Autodesk Inventor part; units mm, degrees
(part 4 of 6)
  line L2681 (34.7928, 6.3295) -> (34.8431, 6.2385)
  line L2682 (34.8431, 6.2385) -> (34.8956, 6.1628)
  line L2683 (34.8956, 6.1628) -> (34.9493, 6.1023)
  line L2684 (34.9493, 6.1023) -> (35.003, 6.0571)
  line L2685 (35.003, 6.0571) -> (35.0554, 6.0269)
  line L2686 (35.0554, 6.0269) -> (35.0808, 6.0175)
  line L2687 (35.0808, 6.0175) -> (35.1054, 6.0117)
  line L2688 (35.1054, 6.0117) -> (35.1292, 6.0095)
  line L2689 (35.1292, 6.0095) -> (35.1519, 6.011)
  line L2690 (35.1519, 6.011) -> (35.1787, 6.0178)
  line L2691 (35.1787, 6.0178) -> (35.427, 6.1078)
  line L2692 (35.427, 6.1078) -> (35.5068, 6.1343)
  line L2693 (35.5068, 6.1343) -> (35.587, 6.1598)
  line L2694 (35.587, 6.1598) -> (35.8408, 6.2329)
  line L2695 (35.8408, 6.2329) -> (35.8665, 6.2431)
  line L2696 (35.8665, 6.2431) -> (35.8857, 6.2553)
  line L2697 (35.8857, 6.2553) -> (35.9037, 6.271)
  line L2698 (35.9037, 6.271) -> (35.9202, 6.2902)
  line L2699 (35.9202, 6.2902) -> (35.9352, 6.3128)
  line L2700 (35.9352, 6.3128) -> (35.9599, 6.368)
  line L2701 (35.9599, 6.368) -> (35.9767, 6.4361)
  line L2702 (35.9767, 6.4361) -> (35.9846, 6.5166)
  line L2703 (35.9846, 6.5166) -> (35.9826, 6.6088)
  line L2704 (35.9826, 6.6088) -> (35.9698, 6.7119)
  line L2705 (35.9698, 6.7119) -> (35.9451, 6.8253)
  line L2706 (35.9451, 6.8253) -> (35.9303, 6.8806)
  line L2707 (35.9303, 6.8806) -> (35.9204, 6.982)
  line L2708 (35.9204, 6.982) -> (35.9201, 7.1118)
  line L2709 (35.9201, 7.1118) -> (35.925, 7.1945)
  line L2710 (35.925, 7.1945) -> (35.9346, 7.2899)
  line L2711 (35.9346, 7.2899) -> (35.9499, 7.3968)
  line L2712 (35.9499, 7.3968) -> (35.9719, 7.5149)
  line L2713 (35.9719, 7.5149) -> (36.0023, 7.6468)
  line L2714 (36.0023, 7.6468) -> (36.0404, 7.7856)
  line L2715 (36.0404, 7.7856) -> (36.0885, 7.9358)
  line L2716 (36.0885, 7.9358) -> (36.147, 8.0951)
  line L2717 (36.147, 8.0951) -> (36.217, 8.2637)
  line L2718 (36.217, 8.2637) -> (36.286, 8.4128)
  arc A83 (36.9384, 8.4814) -> (36.286, 8.4128) centre (37.5, 0) ccw
  line L2719 (36.9384, 8.4814) -> (37.0368, 8.3499)
  line L2720 (37.0368, 8.3499) -> (37.1404, 8.1995)
  line L2721 (37.1404, 8.1995) -> (37.2307, 8.0558)
  line L2722 (37.2307, 8.0558) -> (37.309, 7.919)
  line L2723 (37.309, 7.919) -> (37.3751, 7.7911)
  line L2724 (37.3751, 7.7911) -> (37.4323, 7.6684)
  line L2725 (37.4323, 7.6684) -> (37.4783, 7.5575)
  line L2726 (37.4783, 7.5575) -> (37.5155, 7.4561)
  line L2727 (37.5155, 7.4561) -> (37.5448, 7.3648)
  line L2728 (37.5448, 7.3648) -> (37.5667, 7.2849)
  line L2729 (37.5667, 7.2849) -> (37.5935, 7.1579)
  line L2730 (37.5935, 7.1579) -> (37.6048, 7.0566)
  line L2731 (37.6048, 7.0566) -> (37.6018, 6.9994)
  line L2732 (37.6018, 6.9994) -> (37.6013, 6.8834)
  line L2733 (37.6013, 6.8834) -> (37.6102, 6.7798)
  line L2734 (37.6102, 6.7798) -> (37.6274, 6.6893)
  line L2735 (37.6274, 6.6893) -> (37.6519, 6.6122)
  line L2736 (37.6519, 6.6122) -> (37.6825, 6.5491)
  line L2737 (37.6825, 6.5491) -> (37.7181, 6.5002)
  line L2738 (37.7181, 6.5002) -> (37.7375, 6.4812)
  line L2739 (37.7375, 6.4812) -> (37.7576, 6.4659)
  line L2740 (37.7576, 6.4659) -> (37.7784, 6.4543)
  line L2741 (37.7784, 6.4543) -> (37.7998, 6.4463)
  line L2742 (37.7998, 6.4463) -> (37.8271, 6.4417)
  line L2743 (37.8271, 6.4417) -> (38.0905, 6.4229)
  line L2744 (38.0905, 6.4229) -> (38.1742, 6.4147)
  line L2745 (38.1742, 6.4147) -> (38.2578, 6.4054)
  line L2746 (38.2578, 6.4054) -> (38.5194, 6.3689)
  line L2747 (38.5194, 6.3689) -> (38.547, 6.3678)
  line L2748 (38.547, 6.3678) -> (38.5696, 6.3711)
  line L2749 (38.5696, 6.3711) -> (38.5923, 6.3781)
  line L2750 (38.5923, 6.3781) -> (38.6152, 6.3889)
  line L2751 (38.6152, 6.3889) -> (38.6381, 6.4035)
  line L2752 (38.6381, 6.4035) -> (38.6831, 6.4439)
  line L2753 (38.6831, 6.4439) -> (38.7262, 6.4993)
  line L2754 (38.7262, 6.4993) -> (38.7661, 6.5696)
  line L2755 (38.7661, 6.5696) -> (38.8018, 6.6546)
  line L2756 (38.8018, 6.6546) -> (38.832, 6.754)
  line L2757 (38.832, 6.754) -> (38.8557, 6.8676)
  line L2758 (38.8557, 6.8676) -> (38.8646, 6.9242)
  line L2759 (38.8646, 6.9242) -> (38.8968, 7.0209)
  line L2760 (38.8968, 7.0209) -> (38.9493, 7.1396)
  line L2761 (38.9493, 7.1396) -> (38.9874, 7.2131)
  line L2762 (38.9874, 7.2131) -> (39.035, 7.2964)
  line L2763 (39.035, 7.2964) -> (39.0925, 7.3878)
  line L2764 (39.0925, 7.3878) -> (39.1606, 7.4867)
  line L2765 (39.1606, 7.4867) -> (39.242, 7.5949)
  line L2766 (39.242, 7.5949) -> (39.3333, 7.7062)
  line L2767 (39.3333, 7.7062) -> (39.4383, 7.8238)
  line L2768 (39.4383, 7.8238) -> (39.5565, 7.9456)
  line L2769 (39.5565, 7.9456) -> (39.6891, 8.0711)
  line L2770 (39.6891, 8.0711) -> (39.8127, 8.1793)
  arc A84 (40.4366, 7.9766) -> (39.8127, 8.1793) centre (37.5, 0) ccw
  line L2771 (40.4366, 7.9766) -> (40.4731, 7.8164)
  line L2772 (40.4731, 7.8164) -> (40.5065, 7.6369)
  line L2773 (40.5065, 7.6369) -> (40.5306, 7.4689)
  line L2774 (40.5306, 7.4689) -> (40.5464, 7.312)
  line L2775 (40.5464, 7.312) -> (40.5549, 7.1683)
  line L2776 (40.5549, 7.1683) -> (40.5571, 7.033)
  line L2777 (40.5571, 7.033) -> (40.5541, 6.9129)
  line L2778 (40.5541, 6.9129) -> (40.5468, 6.8051)
  line L2779 (40.5468, 6.8051) -> (40.5364, 6.7098)
  line L2780 (40.5364, 6.7098) -> (40.524, 6.628)
  line L2781 (40.524, 6.628) -> (40.4968, 6.501)
  line L2782 (40.4968, 6.501) -> (40.466, 6.4039)
  line L2783 (40.466, 6.4039) -> (40.4399, 6.3528)
  line L2784 (40.4399, 6.3528) -> (40.3923, 6.2471)
  line L2785 (40.3923, 6.2471) -> (40.3583, 6.1489)
  line L2786 (40.3583, 6.1489) -> (40.3372, 6.0591)
  line L2787 (40.3372, 6.0591) -> (40.3282, 5.9788)
  line L2788 (40.3282, 5.9788) -> (40.3305, 5.9086)
  line L2789 (40.3305, 5.9086) -> (40.3431, 5.8495)
  line L2790 (40.3431, 5.8495) -> (40.3531, 5.8243)
  line L2791 (40.3531, 5.8243) -> (40.3653, 5.8021)
  line L2792 (40.3653, 5.8021) -> (40.3796, 5.783)
  line L2793 (40.3796, 5.783) -> (40.3959, 5.7671)
  line L2794 (40.3959, 5.7671) -> (40.4189, 5.7518)
  line L2795 (40.4189, 5.7518) -> (40.6519, 5.6274)
  line L2796 (40.6519, 5.6274) -> (40.725, 5.5859)
  line L2797 (40.725, 5.5859) -> (40.7976, 5.5434)
  line L2798 (40.7976, 5.5434) -> (41.0218, 5.4037)
  line L2799 (41.0218, 5.4037) -> (41.0465, 5.3914)
  line L2800 (41.0465, 5.3914) -> (41.0684, 5.3853)
  line L2801 (41.0684, 5.3853) -> (41.0921, 5.3824)
  line L2802 (41.0921, 5.3824) -> (41.1174, 5.383)
  line L2803 (41.1174, 5.383) -> (41.1443, 5.387)
  line L2804 (41.1443, 5.387) -> (41.2018, 5.4056)
  line L2805 (41.2018, 5.4056) -> (41.2637, 5.4387)
  line L2806 (41.2637, 5.4387) -> (41.3288, 5.4866)
  line L2807 (41.3288, 5.4866) -> (41.3959, 5.5498)
  line L2808 (41.3959, 5.5498) -> (41.464, 5.6283)
  line L2809 (41.464, 5.6283) -> (41.5318, 5.7225)
  line L2810 (41.5318, 5.7225) -> (41.563, 5.7705)
  line L2811 (41.563, 5.7705) -> (41.6317, 5.8458)
  line L2812 (41.6317, 5.8458) -> (41.728, 5.9328)
  line L2813 (41.728, 5.9328) -> (41.7927, 5.9845)
  line L2814 (41.7927, 5.9845) -> (41.87, 6.0412)
  line L2815 (41.87, 6.0412) -> (41.9597, 6.1014)
  line L2816 (41.9597, 6.1014) -> (42.0622, 6.1641)
  line L2817 (42.0622, 6.1641) -> (42.1805, 6.2298)
  line L2818 (42.1805, 6.2298) -> (42.3092, 6.2943)
  line L2819 (42.3092, 6.2943) -> (42.453, 6.359)
  line L2820 (42.453, 6.359) -> (42.6105, 6.4222)
  line L2821 (42.6105, 6.4222) -> (42.7827, 6.4829)
  line L2822 (42.7827, 6.4829) -> (42.9396, 6.5315)
  arc A85 (43.4271, 6.0925) -> (42.9396, 6.5315) centre (37.5, 0) ccw
  line L2823 (43.4271, 6.0925) -> (43.3952, 5.9314)
  line L2824 (43.3952, 5.9314) -> (43.3528, 5.7538)
  line L2825 (43.3528, 5.7538) -> (43.3065, 5.5905)
  line L2826 (43.3065, 5.5905) -> (43.2571, 5.4408)
  line L2827 (43.2571, 5.4408) -> (43.2064, 5.3061)
  line L2828 (43.2064, 5.3061) -> (43.1534, 5.1815)
  line L2829 (43.1534, 5.1815) -> (43.1018, 5.073)
  line L2830 (43.1018, 5.073) -> (43.0513, 4.9775)
  line L2831 (43.0513, 4.9775) -> (43.003, 4.8947)
  line L2832 (43.003, 4.8947) -> (42.9584, 4.825)
  line L2833 (42.9584, 4.825) -> (42.8819, 4.7201)
  line L2834 (42.8819, 4.7201) -> (42.8142, 4.6439)
  line L2835 (42.8142, 4.6439) -> (42.7697, 4.6078)
  line L2836 (42.7697, 4.6078) -> (42.6832, 4.5306)
  line L2837 (42.6832, 4.5306) -> (42.6121, 4.4547)
  line L2838 (42.6121, 4.4547) -> (42.5564, 4.3813)
  line L2839 (42.5564, 4.3813) -> (42.5155, 4.3115)
  line L2840 (42.5155, 4.3115) -> (42.489, 4.2466)
  line L2841 (42.489, 4.2466) -> (42.4765, 4.1874)
  line L2842 (42.4765, 4.1874) -> (42.4754, 4.1603)
  line L2843 (42.4754, 4.1603) -> (42.4775, 4.1351)
  line L2844 (42.4775, 4.1351) -> (42.4828, 4.1118)
  line L2845 (42.4828, 4.1118) -> (42.4912, 4.0906)
  line L2846 (42.4912, 4.0906) -> (42.506, 4.0673)
  line L2847 (42.506, 4.0673) -> (42.6683, 3.8589)
  line L2848 (42.6683, 3.8589) -> (42.7182, 3.7912)
  line L2849 (42.7182, 3.7912) -> (42.7672, 3.7229)
  line L2850 (42.7672, 3.7229) -> (42.9152, 3.5041)
  line L2851 (42.9152, 3.5041) -> (42.9328, 3.4828)
  line L2852 (42.9328, 3.4828) -> (42.9503, 3.4683)
  line L2853 (42.9503, 3.4683) -> (42.9708, 3.456)
  line L2854 (42.9708, 3.456) -> (42.9942, 3.4462)
  line L2855 (42.9942, 3.4462) -> (43.0203, 3.439)
  line L2856 (43.0203, 3.439) -> (43.0804, 3.4326)
  line L2857 (43.0804, 3.4326) -> (43.1504, 3.4376)
  line L2858 (43.1504, 3.4376) -> (43.2294, 3.455)
  line L2859 (43.2294, 3.455) -> (43.3164, 3.4854)
  line L2860 (43.3164, 3.4854) -> (43.4105, 3.5294)
  line L2861 (43.4105, 3.5294) -> (43.5107, 3.5879)
  line L2862 (43.5107, 3.5879) -> (43.5588, 3.6191)
  line L2863 (43.5588, 3.6191) -> (43.6522, 3.6599)
  line L2864 (43.6522, 3.6599) -> (43.7755, 3.7002)
  line L2865 (43.7755, 3.7002) -> (43.8557, 3.7212)
  line L2866 (43.8557, 3.7212) -> (43.9494, 3.7415)
  line L2867 (43.9494, 3.7415) -> (44.0558, 3.76)
  line L2868 (44.0558, 3.76) -> (44.1749, 3.7755)
  line L2869 (44.1749, 3.7755) -> (44.3097, 3.7874)
  line L2870 (44.3097, 3.7874) -> (44.4536, 3.794)
  line L2871 (44.4536, 3.794) -> (44.6112, 3.7947)
  line L2872 (44.6112, 3.7947) -> (44.7808, 3.7883)
  line L2873 (44.7808, 3.7883) -> (44.9628, 3.7738)
  line L2874 (44.9628, 3.7738) -> (45.1259, 3.7543)
  arc A86 (45.3927, 3.155) -> (45.1259, 3.7543) centre (37.5, 0) ccw
  line L2875 (45.3927, 3.155) -> (45.2981, 3.0208)
  line L2876 (45.2981, 3.0208) -> (45.1871, 2.8758)
  line L2877 (45.1871, 2.8758) -> (45.0783, 2.7455)
  line L2878 (45.0783, 2.7455) -> (44.9724, 2.6288)
  line L2879 (44.9724, 2.6288) -> (44.8712, 2.5263)
  line L2880 (44.8712, 2.5263) -> (44.7722, 2.4341)
  line L2881 (44.7722, 2.4341) -> (44.6809, 2.356)
  line L2882 (44.6809, 2.356) -> (44.5959, 2.2893)
  line L2883 (44.5959, 2.2893) -> (44.5181, 2.2332)
  line L2884 (44.5181, 2.2332) -> (44.449, 2.1877)
  line L2885 (44.449, 2.1877) -> (44.3364, 2.123)
  line L2886 (44.3364, 2.123) -> (44.2436, 2.0809)
  line L2887 (44.2436, 2.0809) -> (44.1883, 2.0661)
  line L2888 (44.1883, 2.0661) -> (44.0778, 2.0307)
  line L2889 (44.0778, 2.0307) -> (43.9821, 1.9903)
  line L2890 (43.9821, 1.9903) -> (43.9013, 1.9459)
  line L2891 (43.9013, 1.9459) -> (43.8355, 1.8988)
  line L2892 (43.8355, 1.8988) -> (43.7849, 1.8502)
  line L2893 (43.7849, 1.8502) -> (43.7494, 1.8012)
  line L2894 (43.7494, 1.8012) -> (43.7374, 1.777)
  line L2895 (43.7374, 1.777) -> (43.729, 1.7531)
  line L2896 (43.729, 1.7531) -> (43.7244, 1.7297)
  line L2897 (43.7244, 1.7297) -> (43.7235, 1.7069)
  line L2898 (43.7235, 1.7069) -> (43.7275, 1.6796)
  line L2899 (43.7275, 1.6796) -> (43.7911, 1.4232)
  line L2900 (43.7911, 1.4232) -> (43.8091, 1.341)
  line L2901 (43.8091, 1.341) -> (43.826, 1.2587)
  line L2902 (43.826, 1.2587) -> (43.8722, 0.9986)
  line L2903 (43.8722, 0.9986) -> (43.8797, 0.972)
  line L2904 (43.8797, 0.972) -> (43.8898, 0.9516)
  line L2905 (43.8898, 0.9516) -> (43.9035, 0.9321)
  line L2906 (43.9035, 0.9321) -> (43.9209, 0.9136)
  line L2907 (43.9209, 0.9136) -> (43.9418, 0.8964)
  line L2908 (43.9418, 0.8964) -> (43.9941, 0.8661)
  line L2909 (43.9941, 0.8661) -> (44.0601, 0.8422)
  line L2910 (44.0601, 0.8422) -> (44.1393, 0.8259)
  line L2911 (44.1393, 0.8259) -> (44.2312, 0.8183)
  line L2912 (44.2312, 0.8183) -> (44.3351, 0.8203)
  line L2913 (44.3351, 0.8203) -> (44.4504, 0.8329)
  line L2914 (44.4504, 0.8329) -> (44.507, 0.8419)
  line L2915 (44.507, 0.8419) -> (44.6089, 0.8412)
  line L2916 (44.6089, 0.8412) -> (44.738, 0.8278)
  line L2917 (44.738, 0.8278) -> (44.8197, 0.8144)
  line L2918 (44.8197, 0.8144) -> (44.9136, 0.7948)
  line L2919 (44.9136, 0.7948) -> (45.0183, 0.7684)
  line L2920 (45.0183, 0.7684) -> (45.1335, 0.7342)
  line L2921 (45.1335, 0.7342) -> (45.2615, 0.6902)
  line L2922 (45.2615, 0.6902) -> (45.3956, 0.6378)
  line L2923 (45.3956, 0.6378) -> (45.5398, 0.5742)
  line L2924 (45.5398, 0.5742) -> (45.6922, 0.4994)
  line L2925 (45.6922, 0.4994) -> (45.8526, 0.4122)
  line L2926 (45.8526, 0.4122) -> (45.9936, 0.328)
  arc A87 (45.9936, -0.328) -> (45.9936, 0.328) centre (37.5, 0) ccw
  line L2927 (45.9936, -0.328) -> (45.8526, -0.4122)
  line L2928 (45.8526, -0.4122) -> (45.6922, -0.4994)
  line L2929 (45.6922, -0.4994) -> (45.5398, -0.5742)
  line L2930 (45.5398, -0.5742) -> (45.3956, -0.6378)
  line L2931 (45.3956, -0.6378) -> (45.2615, -0.6902)
  line L2932 (45.2615, -0.6902) -> (45.1335, -0.7342)
  line L2933 (45.1335, -0.7342) -> (45.0183, -0.7684)
  line L2934 (45.0183, -0.7684) -> (44.9136, -0.7948)
  line L2935 (44.9136, -0.7948) -> (44.8197, -0.8144)
  line L2936 (44.8197, -0.8144) -> (44.738, -0.8278)
  line L2937 (44.738, -0.8278) -> (44.6089, -0.8412)
  line L2938 (44.6089, -0.8412) -> (44.507, -0.8419)
  line L2939 (44.507, -0.8419) -> (44.4504, -0.8329)
  line L2940 (44.4504, -0.8329) -> (44.3351, -0.8203)
  line L2941 (44.3351, -0.8203) -> (44.2312, -0.8183)
  line L2942 (44.2312, -0.8183) -> (44.1393, -0.8259)
  line L2943 (44.1393, -0.8259) -> (44.0601, -0.8422)
  line L2944 (44.0601, -0.8422) -> (43.9941, -0.8661)
  line L2945 (43.9941, -0.8661) -> (43.9418, -0.8964)
  line L2946 (43.9418, -0.8964) -> (43.9209, -0.9136)
  line L2947 (43.9209, -0.9136) -> (43.9035, -0.9321)
  line L2948 (43.9035, -0.9321) -> (43.8898, -0.9516)
  line L2949 (43.8898, -0.9516) -> (43.8797, -0.972)
  line L2950 (43.8797, -0.972) -> (43.8722, -0.9986)
  line L2951 (43.8722, -0.9986) -> (43.826, -1.2587)
  line L2952 (43.826, -1.2587) -> (43.8091, -1.341)
  line L2953 (43.8091, -1.341) -> (43.7911, -1.4232)
  line L2954 (43.7911, -1.4232) -> (43.7275, -1.6796)
  line L2955 (43.7275, -1.6796) -> (43.7235, -1.7069)
  line L2956 (43.7235, -1.7069) -> (43.7244, -1.7297)
  line L2957 (43.7244, -1.7297) -> (43.729, -1.7531)
  line L2958 (43.729, -1.7531) -> (43.7374, -1.777)
  line L2959 (43.7374, -1.777) -> (43.7494, -1.8012)
  line L2960 (43.7494, -1.8012) -> (43.7849, -1.8502)
  line L2961 (43.7849, -1.8502) -> (43.8355, -1.8988)
  line L2962 (43.8355, -1.8988) -> (43.9013, -1.9459)
  line L2963 (43.9013, -1.9459) -> (43.9821, -1.9903)
  line L2964 (43.9821, -1.9903) -> (44.0778, -2.0307)
  line L2965 (44.0778, -2.0307) -> (44.1883, -2.0661)
  line L2966 (44.1883, -2.0661) -> (44.2436, -2.0809)
  line L2967 (44.2436, -2.0809) -> (44.3364, -2.123)
  line L2968 (44.3364, -2.123) -> (44.449, -2.1877)
  line L2969 (44.449, -2.1877) -> (44.5181, -2.2332)
  line L2970 (44.5181, -2.2332) -> (44.5959, -2.2893)
  line L2971 (44.5959, -2.2893) -> (44.6809, -2.356)
  line L2972 (44.6809, -2.356) -> (44.7722, -2.4341)
  line L2973 (44.7722, -2.4341) -> (44.8712, -2.5263)
  line L2974 (44.8712, -2.5263) -> (44.9724, -2.6288)
  line L2975 (44.9724, -2.6288) -> (45.0783, -2.7455)
  line L2976 (45.0783, -2.7455) -> (45.1871, -2.8758)
  line L2977 (45.1871, -2.8758) -> (45.2981, -3.0208)
  line L2978 (45.2981, -3.0208) -> (45.3927, -3.155)
  arc A88 (45.1259, -3.7543) -> (45.3927, -3.155) centre (37.5, 0) ccw
  line L2979 (45.1259, -3.7543) -> (44.9628, -3.7738)
  line L2980 (44.9628, -3.7738) -> (44.7808, -3.7883)
  line L2981 (44.7808, -3.7883) -> (44.6112, -3.7947)
  line L2982 (44.6112, -3.7947) -> (44.4536, -3.794)
  line L2983 (44.4536, -3.794) -> (44.3097, -3.7874)
  line L2984 (44.3097, -3.7874) -> (44.1749, -3.7755)
  line L2985 (44.1749, -3.7755) -> (44.0558, -3.76)
  line L2986 (44.0558, -3.76) -> (43.9494, -3.7415)
  line L2987 (43.9494, -3.7415) -> (43.8557, -3.7212)
  line L2988 (43.8557, -3.7212) -> (43.7755, -3.7002)
  line L2989 (43.7755, -3.7002) -> (43.6522, -3.6599)
  line L2990 (43.6522, -3.6599) -> (43.5588, -3.6191)
  line L2991 (43.5588, -3.6191) -> (43.5107, -3.5879)
  line L2992 (43.5107, -3.5879) -> (43.4105, -3.5294)
  line L2993 (43.4105, -3.5294) -> (43.3164, -3.4854)
  line L2994 (43.3164, -3.4854) -> (43.2294, -3.455)
  line L2995 (43.2294, -3.455) -> (43.1504, -3.4376)
  line L2996 (43.1504, -3.4376) -> (43.0804, -3.4326)
  line L2997 (43.0804, -3.4326) -> (43.0203, -3.439)
  line L2998 (43.0203, -3.439) -> (42.9942, -3.4462)
  line L2999 (42.9942, -3.4462) -> (42.9708, -3.456)
  line L3000 (42.9708, -3.456) -> (42.9503, -3.4683)
  line L3001 (42.9503, -3.4683) -> (42.9328, -3.4828)
  line L3002 (42.9328, -3.4828) -> (42.9152, -3.5041)
  line L3003 (42.9152, -3.5041) -> (42.7672, -3.7229)
  line L3004 (42.7672, -3.7229) -> (42.7182, -3.7912)
  line L3005 (42.7182, -3.7912) -> (42.6683, -3.8589)
  line L3006 (42.6683, -3.8589) -> (42.506, -4.0673)
  line L3007 (42.506, -4.0673) -> (42.4912, -4.0906)
  line L3008 (42.4912, -4.0906) -> (42.4828, -4.1118)
  line L3009 (42.4828, -4.1118) -> (42.4775, -4.1351)
  line L3010 (42.4775, -4.1351) -> (42.4754, -4.1603)
  line L3011 (42.4754, -4.1603) -> (42.4765, -4.1874)
  line L3012 (42.4765, -4.1874) -> (42.489, -4.2466)
  line L3013 (42.489, -4.2466) -> (42.5155, -4.3115)
  line L3014 (42.5155, -4.3115) -> (42.5564, -4.3813)
  line L3015 (42.5564, -4.3813) -> (42.6121, -4.4547)
  line L3016 (42.6121, -4.4547) -> (42.6832, -4.5306)
  line L3017 (42.6832, -4.5306) -> (42.7697, -4.6078)
  line L3018 (42.7697, -4.6078) -> (42.8142, -4.6439)
  line L3019 (42.8142, -4.6439) -> (42.8819, -4.7201)
  line L3020 (42.8819, -4.7201) -> (42.9584, -4.825)
  line L3021 (42.9584, -4.825) -> (43.003, -4.8947)
  line L3022 (43.003, -4.8947) -> (43.0513, -4.9775)
  line L3023 (43.0513, -4.9775) -> (43.1018, -5.073)
  line L3024 (43.1018, -5.073) -> (43.1534, -5.1815)
  line L3025 (43.1534, -5.1815) -> (43.2064, -5.3061)
  line L3026 (43.2064, -5.3061) -> (43.2571, -5.4408)
  line L3027 (43.2571, -5.4408) -> (43.3065, -5.5905)
  line L3028 (43.3065, -5.5905) -> (43.3528, -5.7538)
  line L3029 (43.3528, -5.7538) -> (43.3952, -5.9314)
  line L3030 (43.3952, -5.9314) -> (43.4271, -6.0925)
  arc A89 (42.9396, -6.5315) -> (43.4271, -6.0925) centre (37.5, 0) ccw
  line L3031 (42.9396, -6.5315) -> (42.7827, -6.4829)
  line L3032 (42.7827, -6.4829) -> (42.6105, -6.4222)
  line L3033 (42.6105, -6.4222) -> (42.453, -6.359)
  line L3034 (42.453, -6.359) -> (42.3092, -6.2943)
  line L3035 (42.3092, -6.2943) -> (42.1805, -6.2298)
  line L3036 (42.1805, -6.2298) -> (42.0622, -6.1641)
  line L3037 (42.0622, -6.1641) -> (41.9597, -6.1014)
  line L3038 (41.9597, -6.1014) -> (41.87, -6.0412)
  line L3039 (41.87, -6.0412) -> (41.7927, -5.9845)
  line L3040 (41.7927, -5.9845) -> (41.728, -5.9328)
  line L3041 (41.728, -5.9328) -> (41.6317, -5.8458)
  line L3042 (41.6317, -5.8458) -> (41.563, -5.7705)
  line L3043 (41.563, -5.7705) -> (41.5318, -5.7225)
  line L3044 (41.5318, -5.7225) -> (41.464, -5.6283)
  line L3045 (41.464, -5.6283) -> (41.3959, -5.5498)
  line L3046 (41.3959, -5.5498) -> (41.3288, -5.4866)
  line L3047 (41.3288, -5.4866) -> (41.2637, -5.4387)
  line L3048 (41.2637, -5.4387) -> (41.2018, -5.4056)
  line L3049 (41.2018, -5.4056) -> (41.1443, -5.387)
  line L3050 (41.1443, -5.387) -> (41.1174, -5.383)
  line L3051 (41.1174, -5.383) -> (41.0921, -5.3824)
  line L3052 (41.0921, -5.3824) -> (41.0684, -5.3853)
  line L3053 (41.0684, -5.3853) -> (41.0465, -5.3914)
  line L3054 (41.0465, -5.3914) -> (41.0218, -5.4037)
  line L3055 (41.0218, -5.4037) -> (40.7976, -5.5434)
  line L3056 (40.7976, -5.5434) -> (40.725, -5.5859)
  line L3057 (40.725, -5.5859) -> (40.6519, -5.6274)
  line L3058 (40.6519, -5.6274) -> (40.4189, -5.7518)
  line L3059 (40.4189, -5.7518) -> (40.3959, -5.7671)
  line L3060 (40.3959, -5.7671) -> (40.3796, -5.783)
  line L3061 (40.3796, -5.783) -> (40.3653, -5.8021)
  line L3062 (40.3653, -5.8021) -> (40.3531, -5.8243)
  line L3063 (40.3531, -5.8243) -> (40.3431, -5.8495)
  line L3064 (40.3431, -5.8495) -> (40.3305, -5.9086)
  line L3065 (40.3305, -5.9086) -> (40.3282, -5.9788)
  line L3066 (40.3282, -5.9788) -> (40.3372, -6.0591)
  line L3067 (40.3372, -6.0591) -> (40.3583, -6.1489)
  line L3068 (40.3583, -6.1489) -> (40.3923, -6.2471)
  line L3069 (40.3923, -6.2471) -> (40.4399, -6.3528)
  line L3070 (40.4399, -6.3528) -> (40.466, -6.4039)
  line L3071 (40.466, -6.4039) -> (40.4968, -6.501)
  line L3072 (40.4968, -6.501) -> (40.524, -6.628)
  line L3073 (40.524, -6.628) -> (40.5364, -6.7098)
  line L3074 (40.5364, -6.7098) -> (40.5468, -6.8051)
  line L3075 (40.5468, -6.8051) -> (40.5541, -6.9129)
  line L3076 (40.5541, -6.9129) -> (40.5571, -7.033)
  line L3077 (40.5571, -7.033) -> (40.5549, -7.1683)
  line L3078 (40.5549, -7.1683) -> (40.5464, -7.312)
  line L3079 (40.5464, -7.312) -> (40.5306, -7.4689)
  line L3080 (40.5306, -7.4689) -> (40.5065, -7.6369)
  line L3081 (40.5065, -7.6369) -> (40.4731, -7.8164)
  line L3082 (40.4731, -7.8164) -> (40.4366, -7.9766)
  arc A90 (39.8127, -8.1793) -> (40.4366, -7.9766) centre (37.5, 0) ccw
  line L3083 (39.8127, -8.1793) -> (39.6891, -8.0711)
  line L3084 (39.6891, -8.0711) -> (39.5565, -7.9456)
  line L3085 (39.5565, -7.9456) -> (39.4383, -7.8238)
  line L3086 (39.4383, -7.8238) -> (39.3333, -7.7062)
  line L3087 (39.3333, -7.7062) -> (39.242, -7.5949)
  line L3088 (39.242, -7.5949) -> (39.1606, -7.4867)
  line L3089 (39.1606, -7.4867) -> (39.0925, -7.3878)
  line L3090 (39.0925, -7.3878) -> (39.035, -7.2964)
  line L3091 (39.035, -7.2964) -> (38.9874, -7.2131)
  line L3092 (38.9874, -7.2131) -> (38.9493, -7.1396)
  line L3093 (38.9493, -7.1396) -> (38.8968, -7.0209)
  line L3094 (38.8968, -7.0209) -> (38.8646, -6.9242)
  line L3095 (38.8646, -6.9242) -> (38.8557, -6.8676)
  line L3096 (38.8557, -6.8676) -> (38.832, -6.754)
  line L3097 (38.832, -6.754) -> (38.8018, -6.6546)
  line L3098 (38.8018, -6.6546) -> (38.7661, -6.5696)
  line L3099 (38.7661, -6.5696) -> (38.7262, -6.4993)
  line L3100 (38.7262, -6.4993) -> (38.6831, -6.4439)
  line L3101 (38.6831, -6.4439) -> (38.6381, -6.4035)
  line L3102 (38.6381, -6.4035) -> (38.6152, -6.3889)
  line L3103 (38.6152, -6.3889) -> (38.5923, -6.3781)
  line L3104 (38.5923, -6.3781) -> (38.5696, -6.3711)
  line L3105 (38.5696, -6.3711) -> (38.547, -6.3678)
  line L3106 (38.547, -6.3678) -> (38.5194, -6.3689)
  line L3107 (38.5194, -6.3689) -> (38.2578, -6.4054)
  line L3108 (38.2578, -6.4054) -> (38.1742, -6.4147)
  line L3109 (38.1742, -6.4147) -> (38.0905, -6.4229)
  line L3110 (38.0905, -6.4229) -> (37.8271, -6.4417)
  line L3111 (37.8271, -6.4417) -> (37.7998, -6.4463)
  line L3112 (37.7998, -6.4463) -> (37.7784, -6.4543)
  line L3113 (37.7784, -6.4543) -> (37.7576, -6.4659)
  line L3114 (37.7576, -6.4659) -> (37.7375, -6.4812)
  line L3115 (37.7375, -6.4812) -> (37.7181, -6.5002)
  line L3116 (37.7181, -6.5002) -> (37.6825, -6.5491)
  line L3117 (37.6825, -6.5491) -> (37.6519, -6.6122)
  line L3118 (37.6519, -6.6122) -> (37.6274, -6.6893)
  line L3119 (37.6274, -6.6893) -> (37.6102, -6.7798)
  line L3120 (37.6102, -6.7798) -> (37.6013, -6.8834)
  line L3121 (37.6013, -6.8834) -> (37.6018, -6.9994)
  line L3122 (37.6018, -6.9994) -> (37.6048, -7.0566)
  line L3123 (37.6048, -7.0566) -> (37.5935, -7.1579)
  line L3124 (37.5935, -7.1579) -> (37.5667, -7.2849)
  line L3125 (37.5667, -7.2849) -> (37.5448, -7.3648)
  line L3126 (37.5448, -7.3648) -> (37.5155, -7.4561)
  line L3127 (37.5155, -7.4561) -> (37.4783, -7.5575)
  line L3128 (37.4783, -7.5575) -> (37.4323, -7.6684)
  line L3129 (37.4323, -7.6684) -> (37.3751, -7.7911)
  line L3130 (37.3751, -7.7911) -> (37.309, -7.919)
  line L3131 (37.309, -7.919) -> (37.2307, -8.0558)
  line L3132 (37.2307, -8.0558) -> (37.1404, -8.1995)
  line L3133 (37.1404, -8.1995) -> (37.0368, -8.3499)
  line L3134 (37.0368, -8.3499) -> (36.9384, -8.4814)
  arc A91 (36.286, -8.4128) -> (36.9384, -8.4814) centre (37.5, 0) ccw
  line L3135 (36.286, -8.4128) -> (36.217, -8.2637)
  line L3136 (36.217, -8.2637) -> (36.147, -8.0951)
  line L3137 (36.147, -8.0951) -> (36.0885, -7.9358)
  line L3138 (36.0885, -7.9358) -> (36.0404, -7.7856)
  line L3139 (36.0404, -7.7856) -> (36.0023, -7.6468)
  line L3140 (36.0023, -7.6468) -> (35.9719, -7.5149)
  line L3141 (35.9719, -7.5149) -> (35.9499, -7.3968)
  line L3142 (35.9499, -7.3968) -> (35.9346, -7.2899)
  line L3143 (35.9346, -7.2899) -> (35.925, -7.1945)
  line L3144 (35.925, -7.1945) -> (35.9201, -7.1118)
  line L3145 (35.9201, -7.1118) -> (35.9204, -6.982)
  line L3146 (35.9204, -6.982) -> (35.9303, -6.8806)
  line L3147 (35.9303, -6.8806) -> (35.9451, -6.8253)
  line L3148 (35.9451, -6.8253) -> (35.9698, -6.7119)
  line L3149 (35.9698, -6.7119) -> (35.9826, -6.6088)
  line L3150 (35.9826, -6.6088) -> (35.9846, -6.5166)
  line L3151 (35.9846, -6.5166) -> (35.9767, -6.4361)
  line L3152 (35.9767, -6.4361) -> (35.9599, -6.368)
  line L3153 (35.9599, -6.368) -> (35.9352, -6.3128)
  line L3154 (35.9352, -6.3128) -> (35.9202, -6.2902)
  line L3155 (35.9202, -6.2902) -> (35.9037, -6.271)
  line L3156 (35.9037, -6.271) -> (35.8857, -6.2553)
  line L3157 (35.8857, -6.2553) -> (35.8665, -6.2431)
  line L3158 (35.8665, -6.2431) -> (35.8408, -6.2329)
  line L3159 (35.8408, -6.2329) -> (35.587, -6.1598)
  line L3160 (35.587, -6.1598) -> (35.5068, -6.1343)
  line L3161 (35.5068, -6.1343) -> (35.427, -6.1078)
  line L3162 (35.427, -6.1078) -> (35.1787, -6.0178)
  line L3163 (35.1787, -6.0178) -> (35.1519, -6.011)
  line L3164 (35.1519, -6.011) -> (35.1292, -6.0095)
  line L3165 (35.1292, -6.0095) -> (35.1054, -6.0117)
  line L3166 (35.1054, -6.0117) -> (35.0808, -6.0175)
  line L3167 (35.0808, -6.0175) -> (35.0554, -6.0269)
  line L3168 (35.0554, -6.0269) -> (35.003, -6.0571)
  line L3169 (35.003, -6.0571) -> (34.9493, -6.1023)
  line L3170 (34.9493, -6.1023) -> (34.8956, -6.1628)
  line L3171 (34.8956, -6.1628) -> (34.8431, -6.2385)
  line L3172 (34.8431, -6.2385) -> (34.7928, -6.3295)
  line L3173 (34.7928, -6.3295) -> (34.7461, -6.4357)
  line L3174 (34.7461, -6.4357) -> (34.7256, -6.4892)
  line L3175 (34.7256, -6.4892) -> (34.674, -6.5771)
  line L3176 (34.674, -6.5771) -> (34.5979, -6.6822)
  line L3177 (34.5979, -6.6822) -> (34.5454, -6.7463)
  line L3178 (34.5454, -6.7463) -> (34.4815, -6.8178)
  line L3179 (34.4815, -6.8178) -> (34.4063, -6.8953)
  line L3180 (34.4063, -6.8953) -> (34.3191, -6.9779)
  line L3181 (34.3191, -6.9779) -> (34.217, -7.0668)
  line L3182 (34.217, -7.0668) -> (34.1045, -7.1566)
  line L3183 (34.1045, -7.1566) -> (33.9774, -7.2498)
  line L3184 (33.9774, -7.2498) -> (33.8364, -7.3444)
  line L3185 (33.8364, -7.3444) -> (33.6807, -7.4396)
  line L3186 (33.6807, -7.4396) -> (33.5372, -7.5197)
  arc A92 (32.9691, -7.1917) -> (33.5372, -7.5197) centre (37.5, 0) ccw
  line L3187 (32.9691, -7.1917) -> (32.9668, -7.0275)
  line L3188 (32.9668, -7.0275) -> (32.9714, -6.8449)
  line L3189 (32.9714, -6.8449) -> (32.9828, -6.6756)
  line L3190 (32.9828, -6.6756) -> (32.9999, -6.5189)
  line L3191 (32.9999, -6.5189) -> (33.0215, -6.3765)
  line L3192 (33.0215, -6.3765) -> (33.0474, -6.2437)
  line L3193 (33.0474, -6.2437) -> (33.0754, -6.1269)
  line L3194 (33.0754, -6.1269) -> (33.1049, -6.0229)
  line L3195 (33.1049, -6.0229) -> (33.1349, -5.9319)
  line L3196 (33.1349, -5.9319) -> (33.1641, -5.8544)
  line L3197 (33.1641, -5.8544) -> (33.2171, -5.7359)
  line L3198 (33.2171, -5.7359) -> (33.2674, -5.6473)
  line L3199 (33.2674, -5.6473) -> (33.3035, -5.6028)
  line L3200 (33.3035, -5.6028) -> (33.3721, -5.5092)
  line L3201 (33.3721, -5.5092) -> (33.4258, -5.4202)
  line L3202 (33.4258, -5.4202) -> (33.4651, -5.3368)
  line L3203 (33.4651, -5.3368) -> (33.4906, -5.2601)
  line L3204 (33.4906, -5.2601) -> (33.5029, -5.191)
  line L3205 (33.5029, -5.191) -> (33.5028, -5.1306)
  line L3206 (33.5028, -5.1306) -> (33.4983, -5.1038)
  line L3207 (33.4983, -5.1038) -> (33.491, -5.0796)
  line L3208 (33.491, -5.0796) -> (33.481, -5.0579)
  line L3209 (33.481, -5.0579) -> (33.4684, -5.039)
  line L3210 (33.4684, -5.039) -> (33.4491, -5.0192)
  line L3211 (33.4491, -5.0192) -> (33.2469, -4.8492)
  line L3212 (33.2469, -4.8492) -> (33.1841, -4.7933)
  line L3213 (33.1841, -4.7933) -> (33.122, -4.7366)
  line L3214 (33.122, -4.7366) -> (32.9317, -4.5534)
  line L3215 (32.9317, -4.5534) -> (32.9101, -4.5363)
  line L3216 (32.9101, -4.5363) -> (32.8899, -4.5257)
  line L3217 (32.8899, -4.5257) -> (32.8673, -4.518)
  line L3218 (32.8673, -4.518) -> (32.8424, -4.5132)
  line L3219 (32.8424, -4.5132) -> (32.8154, -4.5116)
  line L3220 (32.8154, -4.5116) -> (32.7552, -4.5178)
  line L3221 (32.7552, -4.5178) -> (32.6878, -4.5373)
  line L3222 (32.6878, -4.5373) -> (32.6142, -4.5707)
  line L3223 (32.6142, -4.5707) -> (32.5353, -4.6185)
  line L3224 (32.5353, -4.6185) -> (32.4524, -4.6812)
  line L3225 (32.4524, -4.6812) -> (32.3666, -4.7592)
  line L3226 (32.3666, -4.7592) -> (32.3261, -4.7997)
  line L3227 (32.3261, -4.7997) -> (32.2432, -4.859)
  line L3228 (32.2432, -4.859) -> (32.1309, -4.9241)
  line L3229 (32.1309, -4.9241) -> (32.0569, -4.9613)
  line L3230 (32.0569, -4.9613) -> (31.9695, -5.0006)
  line L3231 (31.9695, -5.0006) -> (31.8692, -5.0408)
  line L3232 (31.8692, -5.0408) -> (31.756, -5.0808)
  line L3233 (31.756, -5.0808) -> (31.6265, -5.1205)
  line L3234 (31.6265, -5.1205) -> (31.4872, -5.1568)
  line L3235 (31.4872, -5.1568) -> (31.3332, -5.1903)
  line L3236 (31.3332, -5.1903) -> (31.1659, -5.2193)
  line L3237 (31.1659, -5.2193) -> (30.9849, -5.243)
  line L3238 (30.9849, -5.243) -> (30.8213, -5.2578)
  arc A93 (30.4357, -4.7271) -> (30.8213, -5.2578) centre (37.5, 0) ccw
  line L3239 (30.4357, -4.7271) -> (30.5004, -4.5761)
  line L3240 (30.676, 2.741) -> (30.453, 2.6211)
  line L3241 (30.453, 2.6211) -> (30.2376, 2.5111)
  line L3242 (30.2376, 2.5111) -> (30.0323, 2.4116)
  line L3243 (30.0323, 2.4116) -> (29.8355, 2.3213)
  line L3244 (29.8355, 2.3213) -> (29.6473, 2.2396)
  line L3245 (29.6473, 2.2396) -> (29.4705, 2.1673)
  line L3246 (29.4705, 2.1673) -> (29.3033, 2.1029)
  line L3247 (29.3033, 2.1029) -> (28.9724, 1.9849)
  line L3248 (28.9724, 1.9849) -> (28.931, 1.9629)
  line L3249 (28.931, 1.9629) -> (28.9033, 1.9404)
  line L3250 (28.9033, 1.9404) -> (28.8892, 1.9178)
  line L3251 (28.8892, 1.9178) -> (28.8876, 1.9012)
  line L3252 (28.8876, 1.9012) -> (28.9103, 1.5151)
  line L3253 (28.9103, 1.5151) -> (28.9281, 1.1288)
  line L3254 (28.9281, 1.1288) -> (28.9314, 1.1124)
  line L3255 (28.9314, 1.1124) -> (28.9478, 1.0915)
  line L3256 (28.9478, 1.0915) -> (28.9777, 1.0719)
  line L3257 (28.9777, 1.0719) -> (29.0211, 1.0544)
  line L3258 (29.0211, 1.0544) -> (29.3626, 0.9717)
  line L3259 (29.3626, 0.9717) -> (29.5356, 0.9251)
  line L3260 (29.5356, 0.9251) -> (29.719, 0.8717)
  line L3261 (29.719, 0.8717) -> (29.9147, 0.8101)
  line L3262 (29.9147, 0.8101) -> (30.1199, 0.7408)
  line L3263 (30.1199, 0.7408) -> (30.3344, 0.6634)
  line L3264 (30.3344, 0.6634) -> (30.5601, 0.5765)
  line L3265 (30.5601, 0.5765) -> (30.7945, 0.4805)
  line L3266 (30.7945, 0.4805) -> (30.9975, 0.3928)
  arc A94 (30.9975, -0.3928) -> (30.9975, 0.3928) centre (0, 0) ccw
  line L3267 (30.9975, -0.3928) -> (30.7945, -0.4805)
  line L3268 (30.7945, -0.4805) -> (30.5601, -0.5765)
  line L3269 (30.5601, -0.5765) -> (30.3344, -0.6634)
  line L3270 (30.3344, -0.6634) -> (30.1199, -0.7408)
  line L3271 (30.1199, -0.7408) -> (29.9147, -0.8101)
  line L3272 (29.9147, -0.8101) -> (29.719, -0.8717)
  line L3273 (29.719, -0.8717) -> (29.5356, -0.9251)
  line L3274 (29.5356, -0.9251) -> (29.3626, -0.9717)
  line L3275 (29.3626, -0.9717) -> (29.0211, -1.0544)
  line L3276 (29.0211, -1.0544) -> (28.9777, -1.0719)
  line L3277 (28.9777, -1.0719) -> (28.9478, -1.0915)
  line L3278 (28.9478, -1.0915) -> (28.9314, -1.1124)
  line L3279 (28.9314, -1.1124) -> (28.9281, -1.1288)
  line L3280 (28.9281, -1.1288) -> (28.9103, -1.5151)
  line L3281 (28.9103, -1.5151) -> (28.8876, -1.9012)
  line L3282 (28.8876, -1.9012) -> (28.8892, -1.9178)
  line L3283 (28.8892, -1.9178) -> (28.9033, -1.9404)
  line L3284 (28.9033, -1.9404) -> (28.931, -1.9629)
  line L3285 (28.931, -1.9629) -> (28.9724, -1.9849)
  line L3286 (28.9724, -1.9849) -> (29.3033, -2.1029)
  line L3287 (29.3033, -2.1029) -> (29.4705, -2.1673)
  line L3288 (29.4705, -2.1673) -> (29.6473, -2.2396)
  line L3289 (29.6473, -2.2396) -> (29.8355, -2.3213)
  line L3290 (29.8355, -2.3213) -> (30.0323, -2.4116)
  line L3291 (30.0323, -2.4116) -> (30.2376, -2.5111)
  line L3292 (30.2376, -2.5111) -> (30.453, -2.6211)
  line L3293 (30.453, -2.6211) -> (30.676, -2.741)
  line L3294 (30.676, -2.741) -> (30.8688, -2.8495)
  arc A95 (30.7866, -3.6308) -> (30.8688, -2.8495) centre (0, 0) ccw
  line L3295 (30.7866, -3.6308) -> (30.5755, -3.6968)
  line L3296 (30.5755, -3.6968) -> (30.3325, -3.7677)
  line L3297 (30.3325, -3.7677) -> (30.0989, -3.8305)
  line L3298 (30.0989, -3.8305) -> (29.8774, -3.8852)
  line L3299 (29.8774, -3.8852) -> (29.6661, -3.9326)
  line L3300 (29.6661, -3.9326) -> (29.465, -3.9734)
  line L3301 (29.465, -3.9734) -> (29.2771, -4.0074)
  line L3302 (29.2771, -4.0074) -> (29.1001, -4.0356)
  line L3303 (29.1001, -4.0356) -> (28.7519, -4.0822)
  line L3304 (28.7519, -4.0822) -> (28.7069, -4.0951)
  line L3305 (28.7069, -4.0951) -> (28.6751, -4.1114)
  line L3306 (28.6751, -4.1114) -> (28.6567, -4.1305)
  line L3307 (28.6567, -4.1305) -> (28.6516, -4.1464)
  line L3308 (28.6516, -4.1464) -> (28.5936, -4.5288)
  line L3309 (28.5936, -4.5288) -> (28.5306, -4.9104)
  line L3310 (28.5306, -4.9104) -> (28.5305, -4.927)
  line L3311 (28.5305, -4.927) -> (28.5421, -4.951)
  line L3312 (28.5421, -4.951) -> (28.5674, -4.9763)
  line L3313 (28.5674, -4.9763) -> (28.6062, -5.0025)
  line L3314 (28.6062, -5.0025) -> (28.9229, -5.1544)
  line L3315 (28.9229, -5.1544) -> (29.0826, -5.2359)
  line L3316 (29.0826, -5.2359) -> (29.2508, -5.3263)
  line L3317 (29.2508, -5.3263) -> (29.4294, -5.4272)
  line L3318 (29.4294, -5.4272) -> (29.6157, -5.5376)
  line L3319 (29.6157, -5.5376) -> (29.8094, -5.658)
  line L3320 (29.8094, -5.658) -> (30.0122, -5.79)
  line L3321 (30.0122, -5.79) -> (30.2214, -5.9325)
  line L3322 (30.2214, -5.9325) -> (30.4018, -6.0605)
  arc A96 (30.2385, -6.829) -> (30.4018, -6.0605) centre (0, 0) ccw
  line L3323 (30.2385, -6.829) -> (30.0216, -6.8726)
  line L3324 (30.0216, -6.8726) -> (29.7725, -6.9177)
  line L3325 (29.7725, -6.9177) -> (29.5336, -6.9557)
  line L3326 (29.5336, -6.9557) -> (29.3077, -6.9869)
  line L3327 (29.3077, -6.9869) -> (29.0926, -7.012)
  line L3328 (29.0926, -7.012) -> (28.8883, -7.0315)
  line L3329 (28.8883, -7.0315) -> (28.6979, -7.0457)
  line L3330 (28.6979, -7.0457) -> (28.5189, -7.0553)
  line L3331 (28.5189, -7.0553) -> (28.1677, -7.0652)
  line L3332 (28.1677, -7.0652) -> (28.1216, -7.0733)
  line L3333 (28.1216, -7.0733) -> (28.0883, -7.0862)
  line L3334 (28.0883, -7.0862) -> (28.0679, -7.1033)
  line L3335 (28.0679, -7.1033) -> (28.0612, -7.1186)
  line L3336 (28.0612, -7.1186) -> (27.9636, -7.4928)
  line L3337 (27.9636, -7.4928) -> (27.861, -7.8657)
  line L3338 (27.861, -7.8657) -> (27.8592, -7.8823)
  line L3339 (27.8592, -7.8823) -> (27.8683, -7.9073)
  line L3340 (27.8683, -7.9073) -> (27.8907, -7.9351)
  line L3341 (27.8907, -7.9351) -> (27.9266, -7.9652)
  line L3342 (27.9266, -7.9652) -> (28.2257, -8.1494)
  line L3343 (28.2257, -8.1494) -> (28.3759, -8.2472)
  line L3344 (28.3759, -8.2472) -> (28.5338, -8.3547)
  line L3345 (28.5338, -8.3547) -> (28.7009, -8.4737)
  line L3346 (28.7009, -8.4737) -> (28.8746, -8.603)
  line L3347 (28.8746, -8.603) -> (29.0547, -8.7429)
  line L3348 (29.0547, -8.7429) -> (29.2425, -8.8954)
  line L3349 (29.2425, -8.8954) -> (29.4358, -9.059)
  line L3350 (29.4358, -9.059) -> (29.6018, -9.2052)
  arc A97 (29.359, -9.9523) -> (29.6018, -9.2052) centre (0, 0) ccw
  line L3351 (29.359, -9.9523) -> (29.1388, -9.973)
  line L3352 (29.1388, -9.973) -> (28.8863, -9.9918)
  line L3353 (28.8863, -9.9918) -> (28.6447, -10.0047)
  line L3354 (28.6447, -10.0047) -> (28.4168, -10.0121)
  line L3355 (28.4168, -10.0121) -> (28.2002, -10.0146)
  line L3356 (28.2002, -10.0146) -> (27.995, -10.0127)
  line L3357 (27.995, -10.0127) -> (27.8042, -10.0069)
  line L3358 (27.8042, -10.0069) -> (27.6252, -9.9977)
  line L3359 (27.6252, -9.9977) -> (27.2749, -9.9708)
  line L3360 (27.2749, -9.9708) -> (27.2282, -9.9741)
  line L3361 (27.2282, -9.9741) -> (27.1937, -9.9834)
  line L3362 (27.1937, -9.9834) -> (27.1717, -9.9983)
  line L3363 (27.1717, -9.9983) -> (27.1634, -10.0128)
  line L3364 (27.1634, -10.0128) -> (27.0272, -10.3748)
  line L3365 (27.0272, -10.3748) -> (26.8862, -10.7349)
  line L3366 (26.8862, -10.7349) -> (26.8826, -10.7512)
  line L3367 (26.8826, -10.7512) -> (26.8891, -10.777)
  line L3368 (26.8891, -10.777) -> (26.9085, -10.807)
  line L3369 (26.9085, -10.807) -> (26.941, -10.8407)
  line L3370 (26.941, -10.8407) -> (27.2193, -11.0551)
  line L3371 (27.2193, -11.0551) -> (27.3584, -11.1681)
  line L3372 (27.3584, -11.1681) -> (27.5042, -11.2915)
  line L3373 (27.5042, -11.2915) -> (27.6579, -11.4273)
  line L3374 (27.6579, -11.4273) -> (27.8172, -11.5741)
  line L3375 (27.8172, -11.5741) -> (27.9817, -11.7321)
  line L3376 (27.9817, -11.7321) -> (28.1525, -11.9033)
  line L3377 (28.1525, -11.9033) -> (28.3276, -12.0862)
  line L3378 (28.3276, -12.0862) -> (28.4774, -12.249)
  arc A98 (28.1579, -12.9667) -> (28.4774, -12.249) centre (0, 0) ccw
  line L3379 (28.1579, -12.9667) -> (27.9367, -12.9642)
  line L3380 (27.9367, -12.9642) -> (27.6836, -12.9565)
  line L3381 (27.6836, -12.9565) -> (27.442, -12.9441)
  line L3382 (27.442, -12.9441) -> (27.2145, -12.9276)
  line L3383 (27.2145, -12.9276) -> (26.9989, -12.9075)
  line L3384 (26.9989, -12.9075) -> (26.7951, -12.8841)
  line L3385 (26.7951, -12.8841) -> (26.6059, -12.8584)
  line L3386 (26.6059, -12.8584) -> (26.4288, -12.8305)
  line L3387 (26.4288, -12.8305) -> (26.0833, -12.7672)
  line L3388 (26.0833, -12.7672) -> (26.0365, -12.7656)
  line L3389 (26.0365, -12.7656) -> (26.0012, -12.7712)
  line L3390 (26.0012, -12.7712) -> (25.9777, -12.7837)
  line L3391 (25.9777, -12.7837) -> (25.968, -12.7973)
  line L3392 (25.968, -12.7973) -> (25.7946, -13.143)
  line L3393 (25.7946, -13.143) -> (25.6168, -13.4865)
  line L3394 (25.6168, -13.4865) -> (25.6116, -13.5023)
  line L3395 (25.6116, -13.5023) -> (25.6153, -13.5287)
  line L3396 (25.6153, -13.5287) -> (25.6314, -13.5605)
  line L3397 (25.6314, -13.5605) -> (25.6603, -13.5974)
  line L3398 (25.6603, -13.5974) -> (25.9146, -13.8398)
  line L3399 (25.9146, -13.8398) -> (26.0412, -13.9666)
  line L3400 (26.0412, -13.9666) -> (26.1732, -14.1046)
  line L3401 (26.1732, -14.1046) -> (26.312, -14.2558)
  line L3402 (26.312, -14.2558) -> (26.455, -14.4184)
  line L3403 (26.455, -14.4184) -> (26.602, -14.5927)
  line L3404 (26.602, -14.5927) -> (26.7541, -14.7808)
  line L3405 (26.7541, -14.7808) -> (26.9091, -14.9811)
  line L3406 (26.9091, -14.9811) -> (27.041, -15.1586)
  arc A99 (26.6482, -15.8389) -> (27.041, -15.1586) centre (0, 0) ccw
  line L3407 (26.6482, -15.8389) -> (26.4285, -15.8134)
  line L3408 (26.4285, -15.8134) -> (26.1776, -15.7793)
  line L3409 (26.1776, -15.7793) -> (25.9387, -15.7417)
  line L3410 (25.9387, -15.7417) -> (25.7142, -15.7015)
  line L3411 (25.7142, -15.7015) -> (25.5018, -15.6589)
  line L3412 (25.5018, -15.6589) -> (25.3015, -15.6144)
  line L3413 (25.3015, -15.6144) -> (25.1161, -15.569)
  line L3414 (25.1161, -15.569) -> (24.9429, -15.5228)
  line L3415 (24.9429, -15.5228) -> (24.6058, -15.4237)
  line L3416 (24.6058, -15.4237) -> (24.5595, -15.4172)
  line L3417 (24.5595, -15.4172) -> (24.5238, -15.4191)
  line L3418 (24.5238, -15.4191) -> (24.4991, -15.4291)
  line L3419 (24.4991, -15.4291) -> (24.488, -15.4416)
  line L3420 (24.488, -15.4416) -> (24.2795, -15.7673)
  line L3421 (24.2795, -15.7673) -> (24.0668, -16.0903)
  line L3422 (24.0668, -16.0903) -> (24.0599, -16.1055)
  line L3423 (24.0599, -16.1055) -> (24.0608, -16.1321)
  line L3424 (24.0608, -16.1321) -> (24.0735, -16.1655)
  line L3425 (24.0735, -16.1655) -> (24.0984, -16.2052)
  line L3426 (24.0984, -16.2052) -> (24.326, -16.4728)
  line L3427 (24.326, -16.4728) -> (24.4386, -16.6122)
  line L3428 (24.4386, -16.6122) -> (24.5555, -16.7632)
  line L3429 (24.5555, -16.7632) -> (24.6777, -16.928)
  line L3430 (24.6777, -16.928) -> (24.8029, -17.1047)
  line L3431 (24.8029, -17.1047) -> (24.931, -17.2934)
  line L3432 (24.931, -17.2934) -> (25.0625, -17.4964)
  line L3433 (25.0625, -17.4964) -> (25.1957, -17.7118)
  line L3434 (25.1957, -17.7118) -> (25.3084, -17.9021)
  arc A100 (24.8466, -18.5377) -> (25.3084, -17.9021) centre (0, 0) ccw
  line L3435 (24.8466, -18.5377) -> (24.6308, -18.4893)
  line L3436 (24.6308, -18.4893) -> (24.3848, -18.4292)
  line L3437 (24.3848, -18.4292) -> (24.1511, -18.3668)
  line L3438 (24.1511, -18.3668) -> (23.932, -18.3034)
  line L3439 (23.932, -18.3034) -> (23.7253, -18.2388)
  line L3440 (23.7253, -18.2388) -> (23.5308, -18.1736)
  line L3441 (23.5308, -18.1736) -> (23.3511, -18.1091)
  line L3442 (23.3511, -18.1091) -> (23.1837, -18.045)
  line L3443 (23.1837, -18.045) -> (22.8588, -17.9112)
  line L3444 (22.8588, -17.9112) -> (22.8134, -17.8999)
  line L3445 (22.8134, -17.8999) -> (22.7777, -17.8981)
  line L3446 (22.7777, -17.8981) -> (22.7521, -17.9055)
  line L3447 (22.7521, -17.9055) -> (22.7398, -17.9167)
  line L3448 (22.7398, -17.9167) -> (22.4984, -18.2188)
  line L3449 (22.4984, -18.2188) -> (22.2531, -18.5178)
  line L3450 (22.2531, -18.5178) -> (22.2446, -18.5322)
  line L3451 (22.2446, -18.5322) -> (22.2427, -18.5587)
  line L3452 (22.2427, -18.5587) -> (22.2519, -18.5933)
  line L3453 (22.2519, -18.5933) -> (22.2724, -18.6353)
  line L3454 (22.2724, -18.6353) -> (22.4708, -18.9253)
  line L3455 (22.4708, -18.9253) -> (22.5683, -19.0757)
  line L3456 (22.5683, -19.0757) -> (22.6688, -19.2381)
  line L3457 (22.6688, -19.2381) -> (22.773, -19.4148)
  line L3458 (22.773, -19.4148) -> (22.8791, -19.6036)
  line L3459 (22.8791, -19.6036) -> (22.9867, -19.8047)
  line L3460 (22.9867, -19.8047) -> (23.0963, -20.0203)
  line L3461 (23.0963, -20.0203) -> (23.2063, -20.2484)
  line L3462 (23.2063, -20.2484) -> (23.2985, -20.4495)
  arc A101 (22.7728, -21.0333) -> (23.2985, -20.4495) centre (0, 0) ccw
  line L3463 (22.7728, -21.0333) -> (22.5632, -20.9626)
  line L3464 (22.5632, -20.9626) -> (22.3249, -20.8771)
  line L3465 (22.3249, -20.8771) -> (22.099, -20.7906)
  line L3466 (22.099, -20.7906) -> (21.8877, -20.7047)
  line L3467 (21.8877, -20.7047) -> (21.6889, -20.6189)
  line L3468 (21.6889, -20.6189) -> (21.5022, -20.5336)
  line L3469 (21.5022, -20.5336) -> (21.3302, -20.4507)
  line L3470 (21.3302, -20.4507) -> (21.1705, -20.3695)
  line L3471 (21.1705, -20.3695) -> (20.8614, -20.2025)
  line L3472 (20.8614, -20.2025) -> (20.8174, -20.1865)
  line L3473 (20.8174, -20.1865) -> (20.7821, -20.181)
  line L3474 (20.7821, -20.181) -> (20.7559, -20.1856)
  line L3475 (20.7559, -20.1856) -> (20.7424, -20.1955)
  line L3476 (20.7424, -20.1955) -> (20.4707, -20.4707)
  line L3477 (20.4707, -20.4707) -> (20.1955, -20.7424)
  line L3478 (20.1955, -20.7424) -> (20.1856, -20.7559)
  line L3479 (20.1856, -20.7559) -> (20.181, -20.7821)
  line L3480 (20.181, -20.7821) -> (20.1865, -20.8174)
  line L3481 (20.1865, -20.8174) -> (20.2025, -20.8614)
  line L3482 (20.2025, -20.8614) -> (20.3695, -21.1705)
  line L3483 (20.3695, -21.1705) -> (20.4507, -21.3302)
  line L3484 (20.4507, -21.3302) -> (20.5336, -21.5022)
  line L3485 (20.5336, -21.5022) -> (20.6189, -21.6889)
  line L3486 (20.6189, -21.6889) -> (20.7047, -21.8877)
  line L3487 (20.7047, -21.8877) -> (20.7906, -22.099)
  line L3488 (20.7906, -22.099) -> (20.8771, -22.3249)
  line L3489 (20.8771, -22.3249) -> (20.9626, -22.5632)
  line L3490 (20.9626, -22.5632) -> (21.0333, -22.7728)
  arc A102 (20.4495, -23.2985) -> (21.0333, -22.7728) centre (0, 0) ccw
  line L3491 (20.4495, -23.2985) -> (20.2484, -23.2063)
  line L3492 (20.2484, -23.2063) -> (20.0203, -23.0963)
  line L3493 (20.0203, -23.0963) -> (19.8047, -22.9867)
  line L3494 (19.8047, -22.9867) -> (19.6036, -22.8791)
  line L3495 (19.6036, -22.8791) -> (19.4148, -22.773)
  line L3496 (19.4148, -22.773) -> (19.2381, -22.6688)
  line L3497 (19.2381, -22.6688) -> (19.0757, -22.5683)
  line L3498 (19.0757, -22.5683) -> (18.9253, -22.4708)
  line L3499 (18.9253, -22.4708) -> (18.6353, -22.2724)
  line L3500 (18.6353, -22.2724) -> (18.5933, -22.2519)
  line L3501 (18.5933, -22.2519) -> (18.5587, -22.2427)
  line L3502 (18.5587, -22.2427) -> (18.5322, -22.2446)
  line L3503 (18.5322, -22.2446) -> (18.5178, -22.2531)
  line L3504 (18.5178, -22.2531) -> (18.2188, -22.4984)
  line L3505 (18.2188, -22.4984) -> (17.9167, -22.7398)
  line L3506 (17.9167, -22.7398) -> (17.9055, -22.7521)
  line L3507 (17.9055, -22.7521) -> (17.8981, -22.7777)
  line L3508 (17.8981, -22.7777) -> (17.8999, -22.8134)
  line L3509 (17.8999, -22.8134) -> (17.9112, -22.8588)
  line L3510 (17.9112, -22.8588) -> (18.045, -23.1837)
  line L3511 (18.045, -23.1837) -> (18.1091, -23.3511)
  line L3512 (18.1091, -23.3511) -> (18.1736, -23.5308)
  line L3513 (18.1736, -23.5308) -> (18.2388, -23.7253)
  line L3514 (18.2388, -23.7253) -> (18.3034, -23.932)
  line L3515 (18.3034, -23.932) -> (18.3668, -24.1511)
  line L3516 (18.3668, -24.1511) -> (18.4292, -24.3848)
  line L3517 (18.4292, -24.3848) -> (18.4893, -24.6308)
  line L3518 (18.4893, -24.6308) -> (18.5377, -24.8466)
  arc A103 (17.9021, -25.3084) -> (18.5377, -24.8466) centre (0, 0) ccw
  line L3519 (17.9021, -25.3084) -> (17.7118, -25.1957)
  line L3520 (17.7118, -25.1957) -> (17.4964, -25.0625)
  line L3521 (17.4964, -25.0625) -> (17.2934, -24.931)
  line L3522 (17.2934, -24.931) -> (17.1047, -24.8029)
  line L3523 (17.1047, -24.8029) -> (16.928, -24.6777)
  line L3524 (16.928, -24.6777) -> (16.7632, -24.5555)
  line L3525 (16.7632, -24.5555) -> (16.6122, -24.4386)
  line L3526 (16.6122, -24.4386) -> (16.4728, -24.326)
  line L3527 (16.4728, -24.326) -> (16.2052, -24.0984)
  line L3528 (16.2052, -24.0984) -> (16.1655, -24.0735)
  line L3529 (16.1655, -24.0735) -> (16.1321, -24.0608)
  line L3530 (16.1321, -24.0608) -> (16.1055, -24.0599)
  line L3531 (16.1055, -24.0599) -> (16.0903, -24.0668)
  line L3532 (16.0903, -24.0668) -> (15.7673, -24.2795)
  line L3533 (15.7673, -24.2795) -> (15.4416, -24.488)
  line L3534 (15.4416, -24.488) -> (15.4291, -24.4991)
  line L3535 (15.4291, -24.4991) -> (15.4191, -24.5238)
  line L3536 (15.4191, -24.5238) -> (15.4172, -24.5595)
  line L3537 (15.4172, -24.5595) -> (15.4237, -24.6058)
  line L3538 (15.4237, -24.6058) -> (15.5228, -24.9429)
  line L3539 (15.5228, -24.9429) -> (15.569, -25.1161)
  line L3540 (15.569, -25.1161) -> (15.6144, -25.3015)
  line L3541 (15.6144, -25.3015) -> (15.6589, -25.5018)
  line L3542 (15.6589, -25.5018) -> (15.7015, -25.7142)
  line L3543 (15.7015, -25.7142) -> (15.7417, -25.9387)
  line L3544 (15.7417, -25.9387) -> (15.7793, -26.1776)
  line L3545 (15.7793, -26.1776) -> (15.8134, -26.4285)
  line L3546 (15.8134, -26.4285) -> (15.8389, -26.6482)
  arc A104 (15.1586, -27.041) -> (15.8389, -26.6482) centre (0, 0) ccw
  line L3547 (15.1586, -27.041) -> (14.9811, -26.9091)
  line L3548 (14.9811, -26.9091) -> (14.7808, -26.7541)
  line L3549 (14.7808, -26.7541) -> (14.5927, -26.602)
  line L3550 (14.5927, -26.602) -> (14.4184, -26.455)
  line L3551 (14.4184, -26.455) -> (14.2558, -26.312)
  line L3552 (14.2558, -26.312) -> (14.1046, -26.1732)
  line L3553 (14.1046, -26.1732) -> (13.9666, -26.0412)
  line L3554 (13.9666, -26.0412) -> (13.8398, -25.9146)
  line L3555 (13.8398, -25.9146) -> (13.5974, -25.6603)
  line L3556 (13.5974, -25.6603) -> (13.5605, -25.6314)
  line L3557 (13.5605, -25.6314) -> (13.5287, -25.6153)
  line L3558 (13.5287, -25.6153) -> (13.5023, -25.6116)
  line L3559 (13.5023, -25.6116) -> (13.4865, -25.6168)
  line L3560 (13.4865, -25.6168) -> (13.143, -25.7946)
  line L3561 (13.143, -25.7946) -> (12.7973, -25.968)
  line L3562 (12.7973, -25.968) -> (12.7837, -25.9777)
  line L3563 (12.7837, -25.9777) -> (12.7712, -26.0012)
  line L3564 (12.7712, -26.0012) -> (12.7656, -26.0365)
  line L3565 (12.7656, -26.0365) -> (12.7672, -26.0833)
  line L3566 (12.7672, -26.0833) -> (12.8305, -26.4288)
  line L3567 (12.8305, -26.4288) -> (12.8584, -26.6059)
  line L3568 (12.8584, -26.6059) -> (12.8841, -26.7951)
  line L3569 (12.8841, -26.7951) -> (12.9075, -26.9989)
  line L3570 (12.9075, -26.9989) -> (12.9276, -27.2145)
  line L3571 (12.9276, -27.2145) -> (12.9441, -27.442)
  line L3572 (12.9441, -27.442) -> (12.9565, -27.6836)
  line L3573 (12.9565, -27.6836) -> (12.9642, -27.9367)
  line L3574 (12.9642, -27.9367) -> (12.9667, -28.1579)
  arc A105 (12.249, -28.4774) -> (12.9667, -28.1579) centre (0, 0) ccw
  line L3575 (12.249, -28.4774) -> (12.0862, -28.3276)
  line L3576 (12.0862, -28.3276) -> (11.9033, -28.1525)
  line L3577 (11.9033, -28.1525) -> (11.7321, -27.9817)
  line L3578 (11.7321, -27.9817) -> (11.5741, -27.8172)
  line L3579 (11.5741, -27.8172) -> (11.4273, -27.6579)
  line L3580 (11.4273, -27.6579) -> (11.2915, -27.5042)
  line L3581 (11.2915, -27.5042) -> (11.1681, -27.3584)
  line L3582 (11.1681, -27.3584) -> (11.0551, -27.2193)